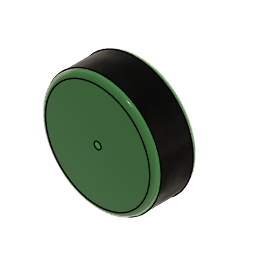
Roues v23 (Autodesk Fusion 360 design; units mm, degrees)
Autodesk Fusion 360 part; units mm, degrees
sketch "Esquisse1" plane through (0, 0, 0) normal (0, 1, 0) x (1, 0, 0)
  circle A0 centre (0, 0) radius 20
  circle A1 centre (0, 0) radius 3.1
  line L0 (-2.1, -2.2804) -> (-2.1, 2.2804)
  line L1 (2.1, -2.2804) -> (2.1, 2.2804)
  line L2 (0, 0) -> (0, -3.1) construction
  line L3 (0, 0) -> (0, 3.1) construction
  dimension "d1" = 40
  dimension "d4" = 6.2
  dimension "d5" = 4.2
  constraint coincident A0.centre A1.centre
  constraint concentric A0 A1
  constraint coincident A1 L0.start
  constraint coincident A1 L0.end
  constraint vertical L0
  constraint coincident A1 L1.start
  constraint coincident A1 L1.end
  constraint parallel L0 L1
  constraint coincident A1 L2.end
  constraint parallel L1 L2
  constraint coincident A1 L3.end
  constraint parallel L2 L3
  constraint symmetric L0 L1 L2
  measures "d1" diameter of A0
  measures "d4" diameter of A1
  measures "d5" distance of L0 L1
extrude "Extrusion1" add sketch "Esquisse1" along normal blind 7 contours A0 | A1 L1 | A1 L0
sketch "Esquisse2" plane through (0, 0, 0) normal (0, -1, 0) x (1, 0, 0)
  arc A0 (2.1, 2.2804) -> (-2.1, 2.2804) centre (0, 0) ccw
  line L0 (2.1, 2.2804) -> (2.1, -2.2804)
  arc A1 (-2.1, -2.2804) -> (2.1, -2.2804) centre (0, 0) ccw
  line L1 (-2.1, -2.2804) -> (-2.1, 2.2804)
  circle A2 centre (0, 0) radius 20
  constraint coincident A0.centre A1.centre
extrude "Extrusion2" add sketch "Esquisse2" against normal blind 4 contours A0 L0 A1 L1
hole "Perçage1" at (0, 0, 0) direction (0, 1, 0) diameter 2.4 depth 23 tip angle 118
sketch "Esquisse3" plane through (0, 7, 0) normal (0, 1, 0) x (-1, 0, 0)
  arc A0 (2.1, 2.2804) -> (-2.1, 2.2804) centre (0, 0) ccw
  line L0 (2.1, 2.2804) -> (2.1, -2.2804)
  arc A1 (-2.1, -2.2804) -> (2.1, -2.2804) centre (0, 0) ccw
  line L1 (-2.1, -2.2804) -> (-2.1, 2.2804)
  circle A2 centre (0, 0) radius 20
  arc A3 (2.1, 2.2804) -> (-2.1, 2.2804) centre (0, 0) ccw
  line L2 (-2.1, 2.2804) -> (-2.1, -2.2804)
  arc A4 (-2.1, -2.2804) -> (2.1, -2.2804) centre (0, 0) ccw
  line L3 (2.1, -2.2804) -> (2.1, 2.2804)
  arc A5 (-3.1, -2.6833) -> (3.1, -2.6833) centre (0, 0) ccw
  line L4 (3.1, 2.6833) -> (3.1, -2.6833)
  arc A6 (3.1, 2.6833) -> (-3.1, 2.6833) centre (0, 0) ccw
  line L5 (-3.1, -2.6833) -> (-3.1, 2.6833)
  circle A7 centre (0, 0) radius 1.2
  dimension "d11" = -1
extrude "Extrusion3" add sketch "Esquisse3" along normal blind 6 contours A5 L4 A6 L5
fillet "Congé1" radius 2 4 edges at (3.1, 10, 2.6833) (3.1, 10, -2.6833) (-3.1, 10, 2.6833) (-3.1, 10, -2.6833)
fillet "Congé2" radius 6 8 edges at (3.1, 7, 0) (2.8457, 7, 2.7648) (0, 7, 4.1) (-2.8457, 7, 2.7648) (-3.1, 7, 0) (-2.8457, 7, -2.7648) (0, 7, -4.1) (2.8457, 7, -2.7648)
sketch "Esquisse4" plane through (0, 7, 0) normal (0, 1, 0) x (-1, 0, 0)
  circle A0 centre (0, 0) radius 20
  line L0 (-9.1, -1.7889) -> (-9.1, 1.7889)
  arc A1 (-5.2905, 8.6035) -> (-9.1, 1.7889) centre (-1.1, 1.7889) ccw
  arc A2 (5.2905, 8.6035) -> (-5.2905, 8.6035) centre (0, 0) ccw
  arc A3 (9.1, 1.7889) -> (5.2905, 8.6035) centre (1.1, 1.7889) ccw
  line L1 (9.1, 1.7889) -> (9.1, -1.7889)
  arc A4 (5.2905, -8.6035) -> (9.1, -1.7889) centre (1.1, -1.7889) ccw
  arc A5 (-5.2905, -8.6035) -> (5.2905, -8.6035) centre (0, 0) ccw
  arc A6 (-9.1, -1.7889) -> (-5.2905, -8.6035) centre (-1.1, -1.7889) ccw
  circle A7 centre (0, 0) radius 20
  circle A8 centre (0, 0) radius 10.25
  line L2 (0, 0) -> (0, 20) construction
  line L3 (0, 10.25) -> (0, 20) construction
  circle A9 centre (0, 0) radius 18
  line L4 (2.5, 12) -> (2.5, 16)
  arc A10 (2.5, 16) -> (-2.5, 16) centre (0, 16) ccw
  line L5 (-2.5, 16) -> (-2.5, 12)
  arc A11 (-2.5, 12) -> (2.5, 12) centre (0, 12) ccw
  line L6 (0, 12) -> (0, 16) construction
  arc A12 (-1.5, 12) -> (1.5, 12) centre (0, 12) ccw
  line L7 (1.5, 12) -> (1.5, 16)
  arc A13 (1.5, 16) -> (-1.5, 16) centre (0, 16) ccw
  line L8 (-1.5, 16) -> (-1.5, 12)
  line L9 (-15.9894, 2.5666) -> (-12.1852, 1.3306)
  line L10 (-15.6804, 3.5177) -> (-11.8762, 2.2816)
  arc A14 (-14.7534, 6.3709) -> (-15.6804, 3.5177) centre (-15.2169, 4.9443) ccw
  arc A15 (-14.4444, 7.3219) -> (-15.9894, 2.5666) centre (-15.2169, 4.9443) ccw
  line L11 (-10.6401, 6.0858) -> (-14.4444, 7.3219)
  line L12 (-10.9492, 5.1348) -> (-14.7534, 6.3709)
  arc A16 (-11.8762, 2.2816) -> (-10.9492, 5.1348) centre (-11.4127, 3.7082) ccw
  arc A17 (-12.1852, 1.3306) -> (-10.6401, 6.0858) centre (-11.4127, 3.7082) ccw
  line L13 (-7.382, -14.4137) -> (-5.0309, -11.1777)
  line L14 (-8.191, -13.8259) -> (-5.8399, -10.5899)
  arc A18 (-10.6181, -12.0626) -> (-8.191, -13.8259) centre (-9.4046, -12.9443) ccw
  arc A19 (-11.4271, -11.4748) -> (-7.382, -14.4137) centre (-9.4046, -12.9443) ccw
  line L15 (-9.076, -8.2387) -> (-11.4271, -11.4748)
  line L16 (-8.2669, -8.8265) -> (-10.6181, -12.0626)
  arc A20 (-5.8399, -10.5899) -> (-8.2669, -8.8265) centre (-7.0534, -9.7082) ccw
  arc A21 (-5.0309, -11.1777) -> (-9.076, -8.2387) centre (-7.0534, -9.7082) ccw
  line L17 (11.4271, -11.4748) -> (9.076, -8.2387)
  line L18 (10.6181, -12.0626) -> (8.2669, -8.8265)
  arc A22 (8.191, -13.8259) -> (10.6181, -12.0626) centre (9.4046, -12.9443) ccw
  arc A23 (7.382, -14.4137) -> (11.4271, -11.4748) centre (9.4046, -12.9443) ccw
  line L19 (5.0309, -11.1777) -> (7.382, -14.4137)
  line L20 (5.8399, -10.5899) -> (8.191, -13.8259)
  arc A24 (8.2669, -8.8265) -> (5.8399, -10.5899) centre (7.0534, -9.7082) ccw
  arc A25 (9.076, -8.2387) -> (5.0309, -11.1777) centre (7.0534, -9.7082) ccw
  line L21 (14.4444, 7.3219) -> (10.6401, 6.0858)
  line L22 (14.7534, 6.3709) -> (10.9492, 5.1348)
  arc A26 (15.6804, 3.5177) -> (14.7534, 6.3709) centre (15.2169, 4.9443) ccw
  arc A27 (15.9894, 2.5666) -> (14.4444, 7.3219) centre (15.2169, 4.9443) ccw
  line L23 (12.1852, 1.3306) -> (15.9894, 2.5666)
  line L24 (11.8762, 2.2816) -> (15.6804, 3.5177)
  arc A28 (10.9492, 5.1348) -> (11.8762, 2.2816) centre (11.4127, 3.7082) ccw
  arc A29 (10.6401, 6.0858) -> (12.1852, 1.3306) centre (11.4127, 3.7082) ccw
  dimension "d18" = 20.5
  dimension "d19" = -2
  dimension "d20" = 16
  dimension "d21" = 12
  dimension "d22" = 5
  dimension "d23" = -1
  dimension "d25" = 360
  constraint concentric A7 A8
  constraint coincident A0.centre A2.centre
  constraint coincident A7 L2.end
  constraint vertical L2
  constraint coincident A8 L3.start
  constraint coincident L2 L3.start
  constraint tangent L4 A10
  constraint tangent A10 L5
  constraint parallel L4 L5
  constraint tangent L5 A11
  constraint tangent L4 A11
  constraint coincident L2 A10.centre
  constraint parallel L2 L6
  measures "d18" diameter of A8
  measures "d20" distance of A0.centre A10.centre
  measures "d21" distance of A0.centre A11.centre
  measures "d22" distance of L4 L5
extrude "Extrusion5" add 1 faces at (13.6578, 0, 1.0235) along direction (0, -1, 0) blind 3
extrude "Extrusion6" add 1 faces at (13.6578, -3, 1.0235) along direction (0, -1, 0) blind 5
extrude "Extrusion7" cut 1 faces at (-1.7989, 4, 0.0299) along direction (0, -1, 0) blind 10
fillet "Congé4" radius 2 2 edges at (-18.6465, -8, -7.2323) (-18.6465, 7, 7.2323)
